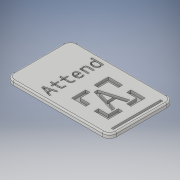
# Autodesk Inventor part: AttendTop
Saved by Autodesk Inventor 2019 (Build 230136000, 136)
## iProperties
Created: 2018-11-13
Part Number: AttendTop
Material: Generic
Document SubType Name: Modeling
Designer: hampu
Density: 1 g/cm^3
Appearance: Default
Author: hampu
Autodesk Inventor part; units mm, degrees
ref_plane "YZ Plane" through (0, 0, 0) normal (1, 0, 0) x (0, 1, 0)
ref_plane "XZ Plane" through (0, 0, 0) normal (0, 1, 0) x (-1, 0, 0)
ref_plane "XY Plane" through (0, 0, 0) normal (0, 0, 1) x (1, 0, 0)
sketch "Sketch1" plane through (0, 0, 0) normal (0, 1, 0) x (-1, 0, 0)
  line L0 (36.595, 22.775) -> (-36.595, 22.775)
  line L1 (-36.595, 22.775) -> (-36.595, -22.775)
  line L2 (-36.595, -22.775) -> (36.595, -22.775)
  line L3 (36.595, -22.775) -> (36.595, 22.775)
  line L4 (36.595, 22.775) -> (-36.595, -22.775) construction
  line L5 (-36.595, 22.775) -> (36.595, -22.775) construction
  line L6 (34.095, -20.275) -> (31.595, -20.275)
  line L7 (31.595, -20.275) -> (31.595, -17.775)
  line L8 (31.595, -17.775) -> (34.095, -17.775)
  line L9 (34.095, -17.775) -> (34.095, -20.275)
  line L10 (34.095, 20.275) -> (31.595, 20.275)
  line L11 (31.595, 20.275) -> (31.595, 17.775)
  line L12 (31.595, 17.775) -> (34.095, 17.775)
  line L13 (34.095, 17.775) -> (34.095, 20.275)
  line L14 (-34.095, 20.275) -> (-31.595, 20.275)
  line L15 (-31.595, 20.275) -> (-31.595, 17.775)
  line L16 (-31.595, 17.775) -> (-34.095, 17.775)
  line L17 (-34.095, 17.775) -> (-34.095, 20.275)
  line L18 (-34.095, -20.275) -> (-31.595, -20.275)
  line L19 (-31.595, -20.275) -> (-31.595, -17.775)
  line L20 (-31.595, -17.775) -> (-34.095, -17.775)
  line L21 (-34.095, -17.775) -> (-34.095, -20.275)
  point P0 (0, 0)
  dimension "d0" = 73.19
  dimension "d1" = 45.55
  dimension "d2" = 2.5
  dimension "d3" = 2.5
  dimension "d4" = 2.5
  dimension "d5" = 2.5
  dimension "d6" = 2.5
  dimension "d7" = 2.5
  dimension "d8" = 2.5
  dimension "d9" = 2.5
  constraints: 44 end point, 10 parallel, 5 horizontal, 5 perpendicular, 2 midpoint
  measures "d0" distance of L2.end L1.end
  measures "d1" distance of L1.end L0.end
  measures "d2" distance of L7.end L8.end
  measures "d3" distance of L6.end L7.end
  measures "d4" distance of L12.end L11.end
  measures "d5" distance of L11.end L10.end
  measures "d6" distance of L15.end L16.end
  measures "d7" distance of L14.end L15.end
  measures "d8" distance of L20.end L19.end
  measures "d9" distance of L19.end L18.end
extrude "Extrusion1" add sketch "Sketch1" along normal blind 3
sketch "Sketch2" plane through (0, 0, 0) normal (0, -1, 0) x (1, 0, 0)
  line L0 (34.095, 17.775) -> (34.095, 20.275) projected
  line L1 (31.595, 17.775) -> (34.095, 17.775) projected
  line L2 (34.095, 20.275) -> (31.595, 20.275)
  line L3 (31.595, 20.275) -> (31.595, 17.775)
  line L4 (31.595, 17.775) -> (34.095, 17.775)
  line L5 (34.095, 17.775) -> (34.095, 20.275)
  line L6 (34.095, -17.775) -> (31.595, -17.775) projected
  line L7 (31.595, -20.275) -> (34.095, -20.275) projected
  line L8 (31.595, -17.775) -> (34.095, -17.775)
  line L9 (34.095, -17.775) -> (34.095, -20.275)
  line L10 (34.095, -20.275) -> (31.595, -20.275)
  line L11 (31.595, -20.275) -> (31.595, -17.775)
  line L12 (-34.095, -20.275) -> (-31.595, -20.275) projected
  line L13 (-31.595, -20.275) -> (-34.095, -20.275)
  line L14 (-34.095, -20.275) -> (-34.095, -17.775)
  line L15 (-34.095, -17.775) -> (-31.595, -17.775)
  line L16 (-31.595, -17.775) -> (-31.595, -20.275)
  line L17 (-34.095, 17.775) -> (-31.595, 17.775) projected
  line L18 (-31.595, 20.275) -> (-34.095, 20.275) projected
  line L19 (-34.095, 17.775) -> (-31.595, 17.775)
  line L20 (-31.595, 17.775) -> (-31.595, 20.275)
  line L21 (-31.595, 20.275) -> (-34.095, 20.275)
  line L22 (-34.095, 20.275) -> (-34.095, 17.775)
  point P0 (0, 0)
  constraints: 32 end point, 8 parallel, 4 horizontal, 4 perpendicular
extrude "Extrusion2" add sketch "Sketch2" along normal blind 3
sketch "Sketch3" plane through (0, 0, 0) normal (0, 1, 0) x (1, 0, 0)
  line L0 (34.095, -20.275) -> (31.595, -20.275) projected
  line L1 (31.595, -17.775) -> (34.095, -17.775) projected
  line L2 (31.595, -20.275) -> (34.095, -20.275)
  line L3 (34.095, -20.275) -> (34.095, -17.775)
  line L4 (34.095, -17.775) -> (31.595, -17.775)
  line L5 (31.595, -17.775) -> (31.595, -20.275)
  line L6 (34.095, 17.775) -> (31.595, 17.775) projected
  line L7 (31.595, 17.775) -> (31.595, 20.275) projected
  line L8 (34.095, 17.775) -> (31.595, 17.775)
  line L9 (31.595, 17.775) -> (31.595, 20.275)
  line L10 (31.595, 20.275) -> (34.095, 20.275)
  line L11 (34.095, 20.275) -> (34.095, 17.775)
  line L12 (-31.595, 20.275) -> (-34.095, 20.275) projected
  line L13 (-31.595, 17.775) -> (-34.095, 17.775) projected
  line L14 (-31.595, 20.275) -> (-34.095, 20.275)
  line L15 (-34.095, 20.275) -> (-34.095, 17.775)
  line L16 (-34.095, 17.775) -> (-31.595, 17.775)
  line L17 (-31.595, 17.775) -> (-31.595, 20.275)
  line L18 (-34.095, -17.775) -> (-34.095, -20.275) projected
  line L19 (-34.095, -17.775) -> (-31.595, -17.775)
  line L20 (-31.595, -17.775) -> (-31.595, -20.275)
  line L21 (-31.595, -20.275) -> (-34.095, -20.275)
  line L22 (-34.095, -20.275) -> (-34.095, -17.775)
  point P0 (0, 0)
  constraints: 32 end point, 8 parallel, 4 horizontal, 4 perpendicular, 2 point on line
extrude "Extrusion3" add sketch "Sketch3" along normal blind 3
sketch "Sketch4" plane through (0, 3, 0) normal (0, 1, 0) x (1, 0, 0)
  line L0 (-36.595, -22.775) -> (36.595, -22.775) projected
  line L1 (36.595, 22.775) -> (-36.595, 22.775) projected
  line L2 (10.8465, 22.775) -> (10.8465, -22.775)
  line L3 (-17.1535, -15.9296) -> (-9.1535, -13.5634)
  line L4 (-9.1535, -13.5634) -> (-9.1535, -14.6197)
  line L5 (-9.1535, -14.6197) -> (-11.738, -15.3803)
  line L6 (-11.738, -15.3803) -> (-11.738, -17.6268)
  line L7 (-11.738, -17.6268) -> (-9.1535, -18.3803)
  line L8 (-9.1535, -18.3803) -> (-9.1535, -19.4296)
  line L9 (-9.1535, -19.4296) -> (-17.1535, -17.0704)
  line L10 (-17.1535, -17.0704) -> (-17.1535, -15.9296)
  line L11 (-12.5408, -17.4155) -> (-12.5408, -15.5845)
  line L12 (-12.5408, -15.5845) -> (-16.0127, -16.4859)
  line L13 (-16.0127, -16.4859) -> (-12.5408, -17.4155)
  line L14 (-14.2873, -10.0704) -> (-11.5267, -10.0704)
  spline S0 degree 2 poles (-11.5267, -10.0704) (-11.0127, -10.0704) (-10.407, -9.9577) (-10.0338, -9.6197) (-9.907, -9.0775) (-9.907, -8.6197) knots 0 0 0 1 2 3 4 4 4
  line L15 (-9.907, -8.6197) -> (-9.907, -7.5423)
  line L16 (-9.907, -7.5423) -> (-9.1535, -7.5915)
  line L17 (-9.1535, -7.5915) -> (-9.1535, -8.5775)
  spline S1 degree 2 poles (-9.1535, -8.5775) (-9.1535, -10.0986) (-9.7098, -10.6056) knots 0 0 0 1 1 1
  spline S2 degree 2 poles (-9.7098, -10.6056) (-10.076, -10.9296) (-10.8859, -11.007) knots 0 0 0 1 1 1
  spline S3 degree 2 poles (-10.8859, -11.007) (-11.2451, -11.0423) (-11.7732, -11.0423) knots 0 0 0 1 1 1
  line L18 (-11.7732, -11.0423) -> (-14.2873, -11.0423)
  line L19 (-14.2873, -11.0423) -> (-14.2873, -12.7113)
  line L20 (-14.2873, -12.7113) -> (-15.0408, -12.5986)
  line L21 (-15.0408, -12.5986) -> (-15.0408, -11.0423)
  line L22 (-15.0408, -11.0423) -> (-17.069, -11.0423)
  line L23 (-17.069, -11.0423) -> (-17.3577, -10.0704)
  line L24 (-17.3577, -10.0704) -> (-15.0408, -10.0704)
  line L25 (-15.0408, -10.0704) -> (-15.0408, -7.5845)
  line L26 (-15.0408, -7.5845) -> (-14.2873, -7.5845)
  line L27 (-14.2873, -7.5845) -> (-14.2873, -10.0704)
  line L28 (-14.2873, -3.4718) -> (-11.5267, -3.4718)
  spline S4 degree 2 poles (-11.5267, -3.4718) (-11.0127, -3.4718) (-10.407, -3.3592) (-10.0338, -3.0211) (-9.907, -2.4789) (-9.907, -2.0211) knots 0 0 0 1 2 3 4 4 4
  line L29 (-9.907, -2.0211) -> (-9.907, -0.9437)
  line L30 (-9.907, -0.9437) -> (-9.1535, -0.993)
  line L31 (-9.1535, -0.993) -> (-9.1535, -1.9789)
  spline S5 degree 2 poles (-9.1535, -1.9789) (-9.1535, -3.5) (-9.7098, -4.007) knots 0 0 0 1 1 1
  spline S6 degree 2 poles (-9.7098, -4.007) (-10.076, -4.331) (-10.8859, -4.4085) knots 0 0 0 1 1 1
  spline S7 degree 2 poles (-10.8859, -4.4085) (-11.2451, -4.4437) (-11.7732, -4.4437) knots 0 0 0 1 1 1
  line L32 (-11.7732, -4.4437) -> (-14.2873, -4.4437)
  line L33 (-14.2873, -4.4437) -> (-14.2873, -6.1127)
  line L34 (-14.2873, -6.1127) -> (-15.0408, -6)
  line L35 (-15.0408, -6) -> (-15.0408, -4.4437)
  line L36 (-15.0408, -4.4437) -> (-17.069, -4.4437)
  line L37 (-17.069, -4.4437) -> (-17.3577, -3.4718)
  line L38 (-17.3577, -3.4718) -> (-15.0408, -3.4718)
  line L39 (-15.0408, -3.4718) -> (-15.0408, -0.9859)
  line L40 (-15.0408, -0.9859) -> (-14.2873, -0.9859)
  line L41 (-14.2873, -0.9859) -> (-14.2873, -3.4718)
  spline S8 degree 2 poles (-9.4282, 2.1972) (-9.8436, 1.5775) (-11.231, 0.9789) (-12.9774, 0.9789) (-14.3718, 1.5352) (-15.2239, 2.6338) (-15.2239, 3.2958) knots 0 0 0 1 2 3 4 5 5 5
  spline S9 degree 2 poles (-15.2239, 3.2958) (-15.2239, 4.5423) (-13.5197, 5.6972) (-12.2732, 5.6972) knots 0 0 0 1 2 2 2
  line L42 (-12.2732, 5.6972) -> (-11.9422, 5.6972)
  line L43 (-11.9422, 5.6972) -> (-11.9422, 1.9718)
  spline S10 degree 2 poles (-11.9422, 1.9718) (-11.0408, 2) (-9.7732, 2.8451) (-9.7732, 3.6901) knots 0 0 0 1 2 2 2
  spline S11 degree 2 poles (-9.7732, 3.6901) (-9.8225, 4.2535) (-10.3859, 5.2606) knots 0 0 0 1 1 1
  line L44 (-10.3859, 5.2606) -> (-9.7169, 5.5845)
  spline S12 degree 2 poles (-9.7169, 5.5845) (-9.0197, 4.8873) (-9.0197, 3.6761) knots 0 0 0 1 1 1
  spline S13 degree 2 poles (-9.0197, 3.6761) (-9.0197, 2.8099) (-9.4282, 2.1972) knots 0 0 0 1 1 1
  spline S14 degree 2 poles (-12.6605, 4.7676) (-14.4704, 4.662) (-14.4704, 3.5) knots 0 0 0 1 1 1
  spline S15 degree 2 poles (-14.4704, 3.5) (-14.4704, 2.1901) (-12.6605, 2) knots 0 0 0 1 1 1
  line L45 (-12.6605, 2) -> (-12.6605, 4.7676)
  spline S16 degree 2 poles (-15.2169, 10.4225) (-15.2169, 12.2535) (-12.9, 12.2535) knots 0 0 0 1 1 1
  line L46 (-12.9, 12.2535) -> (-9.1535, 12.2535)
  line L47 (-9.1535, 12.2535) -> (-9.1535, 11.2817)
  line L48 (-9.1535, 11.2817) -> (-12.7803, 11.2817)
  spline S17 degree 2 poles (-12.7803, 11.2817) (-13.407, 11.2817) (-13.9422, 11.1479) (-14.1113, 11.0211) knots 0 0 0 1 2 2 2
  spline S18 degree 2 poles (-14.1113, 11.0211) (-14.4704, 10.7465) (-14.4704, 10.1268) knots 0 0 0 1 1 1
  spline S19 degree 2 poles (-14.4704, 10.1268) (-14.4704, 9.5) (-13.738, 8.6268) (-13.1394, 8.6268) knots 0 0 0 1 2 2 2
  line L49 (-13.1394, 8.6268) -> (-9.1535, 8.6268)
  line L50 (-9.1535, 8.6268) -> (-9.1535, 7.6479)
  line L51 (-9.1535, 7.6479) -> (-15.0408, 7.6479)
  line L52 (-15.0408, 7.6479) -> (-15.0408, 8.5493)
  line L53 (-15.0408, 8.5493) -> (-14.4, 8.5986)
  spline S20 degree 2 poles (-14.4, 8.5986) (-15.2169, 9.1831) (-15.2169, 10.4225) knots 0 0 0 1 1 1
  line L54 (-14.231, 17.9085) -> (-17.4493, 17.9085)
  line L55 (-17.4493, 17.9085) -> (-17.5549, 18.8873)
  line L56 (-17.5549, 18.8873) -> (-9.1535, 18.8873)
  line L57 (-9.1535, 18.8873) -> (-9.1535, 17.9085)
  line L58 (-9.1535, 17.9085) -> (-10.069, 17.9085)
  spline S21 degree 2 poles (-10.069, 17.9085) (-9.0197, 17.3169) (-9.0197, 16.2254) knots 0 0 0 1 1 1
  spline S22 degree 2 poles (-9.0197, 16.2254) (-9.0197, 14.9789) (-10.8014, 13.8451) (-12.1465, 13.8451) knots 0 0 0 1 2 2 2
  spline S23 degree 2 poles (-12.1465, 13.8451) (-13.7732, 13.8451) (-14.6183, 14.6761) knots 0 0 0 1 1 1
  spline S24 degree 2 poles (-14.6183, 14.6761) (-15.2169, 15.2535) (-15.2169, 16.2324) knots 0 0 0 1 1 1
  spline S25 degree 2 poles (-15.2169, 16.2324) (-15.2169, 16.8944) (-14.6746, 17.7254) (-14.231, 17.9085) knots 0 0 0 1 2 2 2
  spline S26 degree 2 poles (-12.1324, 17.9085) (-13.5056, 17.9085) (-14.4704, 17.0915) (-14.4704, 16.3451) knots 0 0 0 1 2 2 2
  spline S27 degree 2 poles (-14.4704, 16.3451) (-14.4704, 15.3028) (-13.4352, 14.993) knots 0 0 0 1 1 1
  spline S28 degree 2 poles (-13.4352, 14.993) (-12.8718, 14.831) (-12.076, 14.831) knots 0 0 0 1 1 1
  spline S29 degree 2 poles (-12.076, 14.831) (-9.7732, 14.831) (-9.7732, 16.3451) knots 0 0 0 1 1 1
  spline S30 degree 2 poles (-9.7732, 16.3451) (-9.7732, 17.9085) (-12.1324, 17.9085) knots 0 0 0 1 1 1
  point P0 (0, 0)
  constraints: 2 end point, 1 point on line, 1 vertical
extrude "Extrusion4" cut sketch "Sketch4" against normal blind 2
fillet "Fillet1" radius 5 4 edges at (36.595, 1.5, 22.775) (36.595, 1.5, -22.775) (-36.595, 1.5, -22.775) (-36.595, 1.5, 22.775)
fillet "Fillet2" radius 1 8 edges at (0, 3, -22.775) (-35.1305, 3, -21.3105) (-36.595, 3, 0) (-35.1305, 3, 21.3105) (0, 3, 22.775) (35.1305, 3, 21.3105) (36.595, 3, 0) (35.1305, 3, -21.3105)
sketch "Sketch8" plane through (0, 0, 0) normal (0, -1, 0) x (1, 0, 0)
  line L0 (33.995, 17.5) -> (32.495, 17.5)
  line L1 (32.495, 17.5) -> (32.495, -17.5)
  line L2 (32.495, -17.5) -> (33.995, -17.5)
  line L3 (33.995, -17.5) -> (33.995, 17.5)
  line L4 (33.995, 17.5) -> (32.495, -17.5) construction
  line L5 (32.495, 17.5) -> (33.995, -17.5) construction
  point P0 (0, 0)
  point P1 (33.245, 0)
  dimension "d65" = 35
  dimension "d66" = 1.5
  constraints: 12 end point, 2 midpoint, 2 parallel, 1 horizontal, 1 perpendicular
  measures "d65" distance of L1.end L0.end
  measures "d66" distance between parallel lines of L3 L1
extrude "Extrusion8" cut sketch "Sketch8" against normal blind 3
sketch "Sketch9" plane through (0, -3, 0) normal (0, -1, 0) x (1, 0, 0)
  line L0 (-34.095, -17.775) -> (-34.095, -20.275) projected
  line L1 (-31.595, -17.775) -> (-31.595, -20.275) projected
  line L2 (-34.095, -20.275) -> (-31.595, -20.275)
  line L3 (-31.595, -20.275) -> (-31.595, -17.775)
  line L4 (-31.595, -17.775) -> (-34.095, -17.775)
  line L5 (-34.095, -17.775) -> (-34.095, -20.275)
  line L6 (-34.095, 20.275) -> (-31.595, 20.275)
  line L7 (-31.595, 20.275) -> (-31.595, 17.775)
  line L8 (-31.595, 17.775) -> (-34.095, 17.775)
  line L9 (-34.095, 17.775) -> (-34.095, 20.275)
  line L10 (34.095, 20.275) -> (31.595, 20.275) projected
  line L11 (31.595, 20.275) -> (31.595, 17.775) projected
  line L12 (34.095, 20.275) -> (31.595, 20.275)
  line L13 (31.595, 20.275) -> (31.595, 17.775)
  line L14 (31.595, 17.775) -> (34.095, 17.775)
  line L15 (34.095, 17.775) -> (34.095, 20.275)
  line L16 (31.595, -20.275) -> (34.095, -20.275) projected
  line L17 (31.595, -17.775) -> (31.595, -20.275) projected
  line L18 (34.095, -20.275) -> (31.595, -20.275)
  line L19 (31.595, -20.275) -> (31.595, -17.775)
  line L20 (31.595, -17.775) -> (34.095, -17.775)
  line L21 (34.095, -17.775) -> (34.095, -20.275)
  point P0 (0, 0)
  constraints: 32 end point, 8 parallel, 4 horizontal, 4 perpendicular
extrude "Extrusion9" cut sketch "Sketch9" against normal blind 3
sketch "Sketch16" plane through (0, 3, 0) normal (0, 1, 0) x (1, 0, 0)
  line L0 (0, -3) -> (0, -13)
  line L1 (0, -13) -> (10, -13)
  line L2 (10, -13) -> (10, -10)
  line L3 (10, -10) -> (3, -10)
  line L4 (3, -10) -> (3, -3)
  line L5 (3, -3) -> (0, -3)
  line L6 (0, 3) -> (0, 13)
  line L7 (0, 13) -> (10, 13)
  line L8 (10, 13) -> (10, 10)
  line L9 (10, 10) -> (3, 10)
  line L10 (3, 10) -> (3, 3)
  line L11 (3, 3) -> (0, 3)
  line L12 (16, -10) -> (23, -10)
  line L13 (23, -10) -> (23, -3)
  line L14 (23, -3) -> (26, -3)
  line L15 (26, -3) -> (26, -13)
  line L16 (26, -13) -> (16, -13)
  line L17 (16, -13) -> (16, -10)
  line L18 (23, 3) -> (23, 10)
  line L19 (23, 10) -> (16, 10)
  line L20 (16, 10) -> (16, 13)
  line L21 (16, 13) -> (26, 13)
  line L22 (26, 13) -> (26, 3)
  line L23 (26, 3) -> (23, 3)
  line L24 (23, -10) -> (23, 10)
  line L25 (4.25, 1.2401) -> (21.75, 6.4162)
  line L26 (21.75, 6.4162) -> (21.75, 4.1054)
  line L27 (21.75, 4.1054) -> (16.0964, 2.4417)
  line L28 (16.0964, 2.4417) -> (16.0964, -2.4725)
  line L29 (16.0964, -2.4725) -> (21.75, -4.1208)
  line L30 (21.75, -4.1208) -> (21.75, -6.4162)
  line L31 (21.75, -6.4162) -> (4.25, -1.2555)
  line L32 (4.25, -1.2555) -> (4.25, 1.2401)
  line L33 (14.3402, -2.0103) -> (14.3402, 1.9949)
  line L34 (14.3402, 1.9949) -> (6.7456, 0.0231)
  line L35 (6.7456, 0.0231) -> (14.3402, -2.0103)
  point P0 (0, 0)
  dimension "d51" = 10
  dimension "d52" = 10
  dimension "d53" = 3
  dimension "d54" = 7
  dimension "d55" = 10
  dimension "d56" = 10
  dimension "d57" = 3
  dimension "d58" = 7
  dimension "d59" = 7
  dimension "d60" = 7
  dimension "d61" = 3
  constraints: 50 end point, 15 perpendicular, 12 point on line, 2 vertical, 1 horizontal
  measures "d51" distance of L0.start L0.end
  measures "d52" distance of L0.end L1.end
  measures "d53" distance of L1.end L2.end
  measures "d54" distance of L2.end L3.end
  measures "d55" distance of L6.start L6.end
  measures "d56" distance of L6.end L7.end
  measures "d57" distance of L7.end L8.end
  measures "d58" distance of L8.end L9.end
  measures "d59" distance of L12.start L12.end
  measures "d60" distance of L12.end L13.end
  measures "d61" distance of L13.end L14.end
extrude "Extrusion16" cut sketch "Sketch16" against normal blind 2
body "Solid1"
